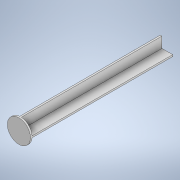
# Autodesk Inventor part: seringa inside
Saved by Autodesk Inventor 2021.2 (Build 252289000, 289)
## iProperties
Created: 2024-04-21
Part Number: seringa inside
Material: Generic
Document SubType Name: Modeling
Designer: cioba
Density: 1 g/cm^3
Appearance: Default
Author: cioba
Autodesk Inventor part; units mm, degrees
ref_plane "YZ Plane" through (0, 0, 0) normal (1, 0, 0) x (0, 1, 0)
ref_plane "XZ Plane" through (0, 0, 0) normal (0, 1, 0) x (-1, 0, 0)
ref_plane "XY Plane" through (0, 0, 0) normal (0, 0, 1) x (1, 0, 0)
sketch "Sketch1" plane through (0, 0, 0) normal (0, 0, 1) x (1, 0, 0)
  line L0 (-1.4564, 16.2472) -> (-1.4564, 9.9656)
  line L1 (-1.4564, 9.9656) -> (-7.738, 9.9656)
  line L2 (-7.738, 8.9656) -> (-1.4564, 8.9656)
  line L3 (-1.4564, 8.9656) -> (-1.4564, 2.684)
  line L4 (-0.4564, 2.684) -> (-0.4564, 8.9656)
  line L5 (-0.4564, 8.9656) -> (5.8252, 8.9656)
  line L6 (5.8252, 9.9656) -> (-0.4564, 9.9656)
  line L7 (-0.4564, 9.9656) -> (-0.4564, 16.2472)
  circle A0 centre (-0.9564, 9.4656) radius 6.8
  constraints: 16 end point, 3 point on line, 1 perpendicular, 1 vertical, 10 other
extrude "Extrusion1" add sketch "Sketch1" against normal blind 83.6 contours A0 L7 L6 L5 L4 L3 L2 L1 L0
extrude "Extrusion2" add sketch "Sketch1" against normal blind 1 contours L0 L1 A0 | A0 L6 L7 | L2 L3 A0 | A0 L4 L5
body "Solid1"
